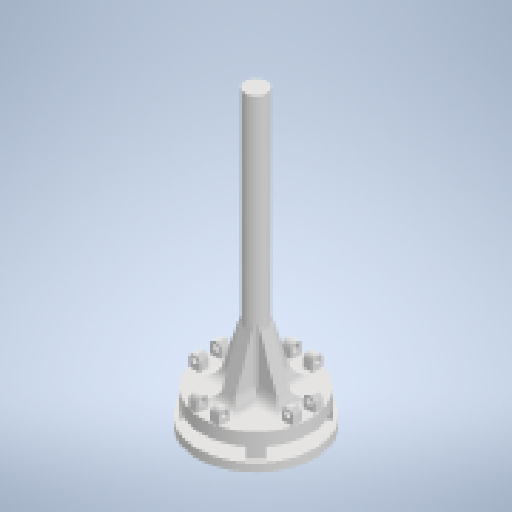
# Autodesk Inventor part: scrambler_vertical_outer
Saved by Autodesk Inventor 2025.2 (Build 292293000, 293)
## iProperties
Created: 2025-10-10
Part Number: scrambler_vertical_outer
Material: Generic
Document SubType Name: Modeling
Designer: pascu
Density: 1 g/cm^3
Appearance: Default
Author: pascu
Autodesk Inventor part; units mm, degrees
ref_plane "YZ Plane" through (0, 0, 0) normal (1, 0, 0) x (0, 1, 0)
ref_plane "XZ Plane" through (0, 0, 0) normal (0, 1, 0) x (-1, 0, 0)
ref_plane "XY Plane" through (0, 0, 0) normal (0, 0, 1) x (1, 0, 0)
sketch "Sketch1" plane through (0, 0, 0) normal (0, 1, 0) x (-1, 0, 0)
  circle A0 centre (0, 0) radius 3.175
  dimension "d0" = 6.35
  constraints: 1 centre point, 1 coincident
  measures "d0" diameter of A0
extrude "Extrusion1" add sketch "Sketch1" along normal blind 76.2
sketch "Sketch2" plane through (0, 0, 0) normal (0, -1, 0) x (1, 0, 0)
  circle A0 centre (0, 0) radius 15.875
  dimension "d3" = 31.75
  constraints: 1 centre point, 1 coincident
  measures "d3" diameter of A0
extrude "Extrusion2" add sketch "Sketch2" along normal blind 9.525
sketch "Sketch4" plane through (0, 0, 0) normal (1, 0, 0) x (0, 1, 0)
  line L0 (0, 0) -> (25.4, 0)
  line L1 (0, 0) -> (0, 8.89)
  line L2 (0, 15.875) -> (0, -15.875) projected
  line L3 (0, 8.89) -> (25.4, 0)
  dimension "d8" = 25.4
  dimension "d9" = 8.89
  constraints: 6 end point, 1 horizontal, 1 point on line
  measures "d8" distance of L0.start L0.end
  measures "d9" distance of L0.start L1.end
extrude "Extrusion3" add sketch "Sketch4" along normal mid plane 3.81
fillet "Fillet1" radius 3.175 1 edges at (0, 0, 8.89)
pattern_circular "Circular Pattern1" count 4 over 360 about axis through (0, 0, 0) along (0, 1, 0) of "Extrusion3", "Fillet1"
fillet "Fillet3" radius 3.175 10 edges at (1.905, 0, 6.8413) (6.8413, 0, 1.905) (6.8413, 0, -1.905) (1.905, 0, -6.8413) (-1.905, 0, -6.8413) (-10.0163, 0, -1.905) (-5.715, 0, -1.905) (-10.0163, 0, 1.905) (-5.715, 0, 1.905) (-1.905, 0, 6.8413)
sketch "Sketch5" plane through (0, 0, 0) normal (1, 0, 0) x (0, 1, 0)
  line L0 (-3.81, 9.525) -> (-6.985, 9.525)
  line L1 (-6.985, 9.525) -> (-6.985, -9.525)
  line L2 (-6.985, -9.525) -> (-3.81, -9.525)
  line L3 (-3.81, -9.525) -> (-3.81, 9.525)
  line L4 (-9.525, 15.875) -> (-9.525, -15.875) projected
  line L5 (0, 15.875) -> (0, -15.875) projected
  point P0 (0, 0)
  point P1 (-6.985, 0)
  point P2 (-9.525, 0)
  dimension "d18" = 3.175
  dimension "d19" = 19.05
  dimension "d20" = 3.81
  constraints: 8 end point, 2 midpoint, 2 parallel, 1 horizontal, 1 horizontal alignment, 1 perpendicular
  measures "d18" distance of L2.end L1.end
  measures "d19" distance of L1.end L0.end
  measures "d20" distance between parallel lines of L5 L3
extrude "Extrusion4" cut sketch "Sketch5" along normal through all both and the other way through all
pattern_circular "Circular Pattern2" count 4 over 360 about axis through (0, 0, 0) along (0, 1, 0) of "Extrusion4"
sketch "Sketch6" plane through (0, 0, 0) normal (0, 1, 0) x (1, 0, 0)
  line L0 (12.0733, 4.445) -> (15.2483, 4.445)
  line L1 (15.2483, 4.445) -> (15.2483, 1.905)
  line L2 (15.2483, -4.445) -> (12.0733, -4.445)
  line L3 (12.0733, -4.445) -> (12.0733, -1.905)
  line L4 (11.1426, -5.08) -> (11.1426, 5.08) projected
  line L5 (15.2483, -1.905) -> (12.0733, -1.905)
  line L6 (12.0733, -1.905) -> (12.0733, 1.905) construction
  line L7 (12.0733, 1.905) -> (15.2483, 1.905)
  line L8 (15.2483, 1.905) -> (15.2483, -1.905) construction
  line L9 (15.2483, 1.905) -> (15.2483, -1.905)
  line L10 (12.0733, 1.905) -> (12.0733, 4.445)
  line L11 (12.0733, -1.905) -> (12.0733, 1.905) construction
  line L12 (15.2483, -1.905) -> (15.2483, -4.445)
  point P0 (0, 0)
  point P1 (11.1426, 0)
  point P2 (11.1426, 0)
  point P3 (11.1426, 0)
  dimension "d26" = 3.175
  dimension "d27" = 8.89
  dimension "d29" = 4.445
  dimension "d30" = 3.81
  dimension "d31" = 1.905
  constraints: 24 end point, 12 parallel, 4 perpendicular, 3 midpoint, 2 horizontal, 1 point on line
  measures "d26" distance of L2.start L2.end
  measures "d27" distance of L0.end L2.start
  measures "d29" distance from line of L2 point (11.143, 0)
  measures "d30" distance of L3.end L6.end
  measures "d31" distance from line of point (11.143, 0) L7
extrude "Extrusion5" add sketch "Sketch6" along normal blind 3.81
fillet "Fillet4" radius 1.5875 4 edges at (15.2483, 3.81, 3.175) (12.0733, 3.81, 3.175) (15.2483, 3.81, -3.175) (12.0733, 3.81, -3.175)
sketch "Sketch7" plane through (12.0733, 0, 4.445) normal (0, 0, 1) x (1, 0, 0)
  arc A0 (3.175, 2.2225) -> (0, 2.2225) centre (1.5875, 2.2225) ccw projected
  point P0 (-12.0733, 0)
  constraints: 1 coincident
hole "Hole1" at (13.6608, 2.2225, 4.445) direction (0, 0, -1) diameter 1.778 end through all
pattern_circular "Circular Pattern3" count 4 over 360 about axis through (0, 0, 0) along (0, 1, 0) of "Extrusion5", "Fillet4", "Hole1"
sketch "Sketch8" plane through (0, -6.985, 0) normal (0, 1, 0) x (1, 0, 0)
  circle A0 centre (0, 0) radius 17.145
  dimension "d45" = 34.29
  constraints: 1 centre point, 1 coincident
  measures "d45" diameter of A0
extrude "Extrusion6" add sketch "Sketch8" against normal blind 2.54
body "Solid1"
